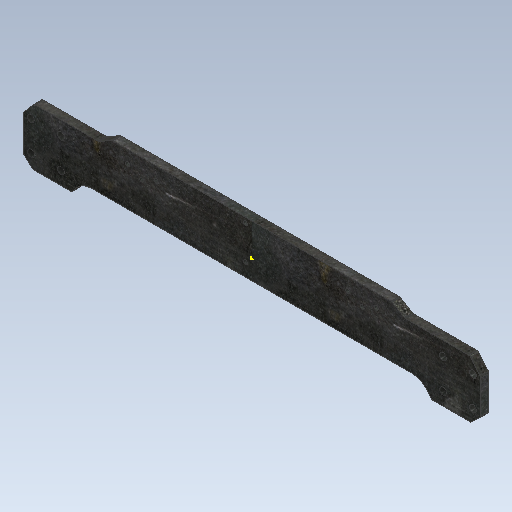
# Autodesk Inventor part: FRONT PLATE P1.2
Saved by Autodesk Inventor 2023 (Build 270158000, 158)
## iProperties
Created: 2019-09-15
Part Number: FRONT PLATE P1.2
Material: Generic
Document SubType Name: Modeling
Designer: pepd9
Density: 1 g/cm^3
Appearance: Plate
Author: pepd9
Autodesk Inventor part; units mm, degrees
ref_plane "YZ Plane" through (0, 0, 0) normal (1, 0, 0) x (0, 1, 0)
ref_plane "XZ Plane" through (0, 0, 0) normal (0, 1, 0) x (-1, 0, 0)
ref_plane "XY Plane" through (0, 0, 0) normal (0, 0, 1) x (1, 0, 0)
sketch "Sketch1" plane through (0, 0, 0) normal (0, 0, 1) x (1, 0, 0)
  line L0 (-176.5, -25) -> (176.5, -25)
  line L1 (176.5, -25) -> (176.5, 25)
  line L2 (176.5, 25) -> (-176.5, 25)
  line L3 (-176.5, 25) -> (-176.5, -25)
  line L4 (-176.5, -25) -> (176.5, 25) construction
  line L5 (176.5, -25) -> (-176.5, 25) construction
  point P0 (0, 0)
  dimension "d0" = 50
  dimension "d1" = 353
  constraints: 12 end point, 2 midpoint, 2 parallel, 1 horizontal, 1 perpendicular
  measures "d0" distance of L2.end L0.start
  measures "d1" distance of L1.end L2.end
extrude "Extrusion1" add sketch "Sketch1" along normal blind 6.35
sketch "Sketch2" plane through (0, 0, 6.35) normal (0, 0, 1) x (1, 0, 0)
  line L0 (-176.5, -25) -> (176.5, -25) projected
  line L1 (-176.5, 25) -> (-176.5, -25) projected
  line L2 (0, 0) -> (0, -33.6266)
  point P0 (-147.4, -15.1)
  point P1 (147.4, -15.1)
  point P2 (-170.6, -15.1)
  point P3 (-147.4, 8.1)
  point P4 (-170.6, 8.1)
  point P5 (170.6, -15.1)
  point P6 (147.4, 8.1)
  point P7 (170.6, 8.1)
  dimension "d4" = 294.8
  dimension "d5" = 147.4
  dimension "d6" = 9.9
  dimension "d9" = 23.2
  dimension "d12" = 23.2
  constraints: 3 symmetric about line, 2 end point, 2 vertical, 1 horizontal, 1 horizontal alignment, 3 other
  measures "d4" distance of point (147.4, -15.1) point (-147.4, -15.1)
  measures "d5" horizontal distance of point (147.4, -15.1) L2.start
  measures "d6" distance from line of L0 point (-147.4, -15.1)
  measures "d9" distance of point (-147.4, -15.1) point (-170.6, -15.1)
  measures "d12" distance of point (-147.4, -15.1) point (-147.4, 8.1)
hole "Hole1" at (-147.4, -15.1, 6.35) at (147.4, -15.1, 6.35) at (-170.6, -15.1, 6.35) at (-147.4, 8.1, 6.35) at (-170.6, 8.1, 6.35) at (170.6, -15.1, 6.35) at (170.6, 8.1, 6.35) at (147.4, 8.1, 6.35) direction (0, 0, -1) diameter 5.4 end through all
chamfer "Chamfer1" distance 7 distance2 7.5 1 edges at (-176.5, -25, 3.175) measured on face at (-176.5, 8.3333, 2.1167)
chamfer "Chamfer2" distance 7 distance2 7.5 1 edges at (176.5, -25, 3.175) measured on face at (176.5, -8.3333, 4.2333)
sketch "Sketch3" plane through (0, 0, 6.35) normal (0, 0, 1) x (1, 0, 0)
  point P0 (0, 0)
sketch "Sketch4" plane through (0, 0, 6.35) normal (0, 0, 1) x (1, 0, 0)
  circle A0 centre (96, 14.9487) radius 1.6 projected
  circle A1 centre (85, 10.04) radius 1.6 projected
  circle A2 centre (74, 14.9487) radius 1.6 projected
  circle A3 centre (-74, 14.9487) radius 1.6 projected
  circle A4 centre (-85, 10.04) radius 1.6 projected
  circle A5 centre (-96, 14.9487) radius 1.6 projected
  point P0 (0, 0)
hole "Hole2" at (-96, 14.9487, 6.35) at (-85, 10.04, 6.35) at (-74, 14.9487, 6.35) at (74, 14.9487, 6.35) at (85, 10.04, 6.35) at (96, 14.9487, 6.35) direction (0, 0, -1) diameter 3.2 end through all
sketch "Sketch5" plane through (0, 0, 6.35) normal (0, 0, 1) x (1, 0, 0)
  circle A0 centre (-5, 21) radius 2.75 projected
  circle A1 centre (-5, -5) radius 2.75 projected
  point P0 (0, 0)
hole "Hole3" at (-5, 21, 6.35) at (-5, -5, 6.35) direction (0, 0, -1) diameter 3.2 end through all
sketch "Sketch6" plane through (0, 0, 6.35) normal (0, 0, 1) x (1, 0, 0)
  line L0 (-176.5, 9) -> (-168.109, 19)
  line L1 (-168.109, 19) -> (-118.109, 19)
  line L2 (-118.109, 19) -> (-107.7167, 25)
  line L3 (176.5, 25) -> (-176.5, 25) projected
  line L4 (-169, -25) -> (169, -25) projected
  line L5 (-139, -25) -> (-130.609, -15)
  line L6 (-130.609, -15) -> (130.609, -15)
  line L7 (130.609, -15) -> (139, -25)
  line L8 (0, 25) -> (0, 0) construction
  line L9 (-176.5, 25) -> (-176.5, -18) projected
  line L10 (176.5, 9) -> (168.109, 19)
  line L11 (168.109, 19) -> (118.109, 19)
  line L12 (118.109, 19) -> (107.7167, 25)
  line L13 (176.5, -18) -> (176.5, 25) projected
  dimension "d42" = 30
  dimension "d43" = 50
  dimension "d44" = 50
  dimension "d45" = 10
  dimension "d46" = 40
  dimension "d47" = 16
  dimension "d48" = 50
  dimension "d49" = 6
  dimension "d52" = 30
  dimension "d53" = 30
  constraints: 20 end point, 4 point on line, 4 symmetric about line, 1 horizontal, 1 parallel, 1 vertical
  measures "d42" angle of L3 L2
  measures "d43" angle of L4 L5
  measures "d44" angle of L4 L7
  measures "d45" distance between parallel lines of L4 L6
  measures "d46" angle of L9 L0
  measures "d47" distance from line of L3 L0.start
  measures "d48" distance of L0.end L1.end
  measures "d49" distance between parallel lines of L3 L1
  measures "d52" distance of L4.start L5.start
  measures "d53" distance of L4.end L7.end
extrude "Extrusion2" cut sketch "Sketch6" against normal blind 10
fillet "Fillet1" radius 15 2 edges at (-130.609, -15, 3.175) (130.609, -15, 3.175)
fillet "Fillet1" radius 2 10 edges at (176.5, -18, 3.175) (176.5, 9, 3.175) (168.109, 19, 3.175) (118.109, 19, 3.175) (107.7167, 25, 3.175) (-118.109, 19, 3.175) (-107.7167, 25, 3.175) (-168.109, 19, 3.175) (-176.5, 9, 3.175) (-176.5, -18, 3.175)
body "Solid1"
